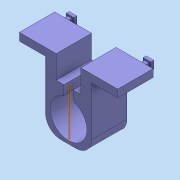
# Autodesk Inventor part: support_codeur
Saved by Autodesk Inventor 2017 (Build 210142000, 142)
## iProperties
Created: 2017-12-27
Part Number: support_codeur
Material: Generic
Document SubType Name: Modeling
Designer: franc
Density: 1 g/cm^3
Appearance: Default
Author: franc
Autodesk Inventor part; units mm, degrees
ref_plane "YZ Plane" through (0, 0, 0) normal (1, 0, 0) x (0, 1, 0)
ref_plane "XZ Plane" through (0, 0, 0) normal (0, 1, 0) x (-1, 0, 0)
ref_plane "XY Plane" through (0, 0, 0) normal (0, 0, 1) x (1, 0, 0)
sketch "Esquisse1" plane through (0, 0, 0) normal (0, 1, 0) x (-1, 0, 0)
  line L0 (7.2872, 10.2128) -> (-22.7128, 10.2128)
  line L1 (-22.7128, 10.2128) -> (-22.7128, -19.7872)
  line L2 (-22.7128, -19.7872) -> (7.2872, -19.7872)
  line L3 (7.2872, -19.7872) -> (7.2872, 10.2128)
  point P0 (0, 0)
  dimension "d0" = 30
  dimension "d1" = 30
  constraints: 8 end point, 2 parallel, 1 horizontal, 1 perpendicular
  measures "d0" distance of L2.end L0.start
  measures "d1" distance of L0.start L0.end
extrude "Extrusion1" add sketch "Esquisse1" along normal blind 23
ref_plane "Plan médian" through (7.7128, 0, 10.2128) normal (1, 0, 0) x (0, 0, -1)
sketch "Esquisse4" plane through (0, 0, 0) normal (0, -1, 0) x (1, 0, 0)
  circle A0 centre (7.7128, -7.8122) radius 11.975 projected
  arc A1 (4.2482, 4.1575) -> (4.0453, 3.779) centre (4.3314, 3.8692) ccw projected
  line L0 (4.1002, 3.6049) -> (4.0453, 3.779)
  line L1 (4.7128, 6.1957) -> (4.7128, 4.2818)
  arc A2 (11.3803, 3.779) -> (11.1773, 4.1575) centre (11.0942, 3.8692) ccw projected
  line L2 (11.3254, 3.6049) -> (11.3803, 3.779)
  line L3 (4.2482, 4.1575) -> (4.7128, 4.2781)
  line L4 (11.1773, 4.1575) -> (10.7128, 4.3039)
  line L5 (4.7128, 4.2818) -> (4.7128, 4.2781)
  line L6 (4.7128, 6.1957) -> (4.7128, 10.2128)
  line L7 (-7.2872, 10.2128) -> (22.7128, 10.2128) projected
  line L8 (10.7128, 5.8358) -> (10.7128, 10.2128)
  line L9 (10.7128, 5.8358) -> (10.7128, 4.3039)
  point P0 (0, 0)
  constraints: 18 end point, 5 point on line, 4 vertical, 3 point on circle, 1 parallel, 6 other
extrude "Extrusion2" cut sketch "Esquisse4" against normal blind 22
sketch "Esquisse5" plane through (0, 22, 0) normal (0, -1, 0) x (1, 0, 0)
  circle A0 centre (15.507, -3.3122) radius 1.25 projected
  circle A1 centre (-0.0815, -3.3122) radius 1.25 projected
  circle A2 centre (7.7128, -16.8122) radius 1.25 projected
  circle A3 centre (7.7128, -7.8122) radius 6 projected
  point P0 (0, 0)
extrude "Extrusion3" cut sketch "Esquisse5" against normal through all
sketch "Esquisse6" plane through (-7.2872, 23, 10.2128) normal (0, 0, 1) x (1, 0, 0)
  line L0 (0, -23) -> (12, -23) projected
  line L1 (5.9558, 0) -> (8.4558, 0) projected
  line L2 (0, -23) -> (7, -23)
  line L3 (7, -23) -> (7, 0)
  line L4 (7, 0) -> (0, 0)
  line L5 (0, 0) -> (0, -23)
  line L6 (30, -23) -> (30, 0) projected
  line L7 (0, 0) -> (30, 0) projected
  line L8 (30, -23) -> (23, -23)
  line L9 (23, -23) -> (23, 0)
  line L10 (23, 0) -> (30, 0)
  line L11 (30, 0) -> (30, -23)
  point P0 (7.2872, -23)
  dimension "d8" = 7
  dimension "d9" = 7
  constraints: 16 end point, 4 parallel, 2 horizontal, 2 perpendicular, 2 point on line
  measures "d8" distance between parallel lines of L5 L3
  measures "d9" distance between parallel lines of L6 L9
extrude "Extrusion4" add sketch "Esquisse6" along normal blind 10
sketch "Esquisse7" plane through (-7.2872, 23, 20.2128) normal (0, 0, 1) x (1, 0, 0)
  line L0 (7, 0) -> (-17, 0)
  line L1 (-17, 0) -> (-17, -23)
  line L2 (-17, -23) -> (7, -23)
  line L3 (7, -23) -> (7, 0)
  line L4 (30, 0) -> (0, 0) projected
  line L5 (23, 0) -> (47, 0)
  line L6 (47, 0) -> (47, -23)
  line L7 (47, -23) -> (23, -23)
  line L8 (23, -23) -> (23, 0)
  line L9 (0, 0) -> (0, -23) projected
  line L10 (30, -23) -> (30, 0) projected
  point P0 (7.2872, -23)
  dimension "d12" = 17
  dimension "d13" = 17
  constraints: 16 end point, 4 parallel, 2 horizontal, 2 perpendicular, 1 point on line
  measures "d12" distance between parallel lines of L1 L9
  measures "d13" distance between parallel lines of L6 L10
extrude "Extrusion5" add sketch "Esquisse7" along normal blind 5
sketch "Esquisse8" plane through (0, 23, 0) normal (0, 1, 0) x (1, 0, 0)
  line L0 (34.2128, -24.2128) -> (31.2128, -24.2128)
  line L1 (31.2128, -24.2128) -> (31.2128, -21.2128)
  line L2 (31.2128, -21.2128) -> (34.2128, -21.2128)
  line L3 (34.2128, -21.2128) -> (34.2128, -24.2128)
  line L4 (39.7128, -20.2128) -> (39.7128, -25.2128) projected
  line L5 (39.7128, -20.2128) -> (22.7128, -20.2128) projected
  line L6 (-16.0084, -24.2128) -> (-18.7872, -24.2128)
  line L7 (-18.7872, -24.2128) -> (-18.7872, -21.2128)
  line L8 (-18.7872, -21.2128) -> (-16.0084, -21.2128)
  line L9 (-16.0084, -21.2128) -> (-16.0084, -24.2128)
  line L10 (-0.2872, -25.2128) -> (-24.2872, -25.2128) projected
  line L11 (-24.2872, -20.2128) -> (-24.2872, -25.2128) projected
  point P0 (0, 0)
  point P1 (-0.4939, -25.2128)
  dimension "d16" = 5.5
  dimension "d17" = 3
  dimension "d18" = 3
  dimension "d19" = 1
  dimension "d20" = 3
  dimension "d21" = 1
  dimension "d22" = 5.5
  constraints: 16 end point, 4 parallel, 2 horizontal, 2 perpendicular
  measures "d16" distance between parallel lines of L4 L3
  measures "d17" distance of L2.end L0.start
  measures "d18" distance of L0.start L0.end
  measures "d19" distance between parallel lines of L5 L2
  measures "d20" distance of L6.end L7.end
  measures "d21" distance between parallel lines of L10 L6
  measures "d22" distance between parallel lines of L11 L7
extrude "Extrusion6" add sketch "Esquisse8" along normal blind 3
sketch "Esquisse9" plane through (0, 26, 0) normal (0, 1, 0) x (1, 0, 0)
  line L0 (15.7128, -25.2128) -> (39.7128, -25.2128) projected
  line L1 (22.7128, -20.2128) -> (39.7128, -20.2128) projected
  line L2 (35.2128, -25.2128) -> (30.2128, -25.2128)
  line L3 (30.2128, -25.2128) -> (30.2128, -20.2128)
  line L4 (30.2128, -20.2128) -> (35.2128, -20.2128)
  line L5 (35.2128, -20.2128) -> (35.2128, -25.2128)
  line L6 (39.7128, -20.2128) -> (39.7128, -25.2128) projected
  line L7 (-24.2872, -25.2128) -> (-0.2872, -25.2128) projected
  line L8 (-14.7872, -25.2128) -> (-19.7872, -25.2128)
  line L9 (-19.7872, -25.2128) -> (-19.7872, -20.2128)
  line L10 (-19.7872, -20.2128) -> (-14.7872, -20.2128)
  line L11 (-14.7872, -20.2128) -> (-14.7872, -25.2128)
  line L12 (-24.2872, -20.2128) -> (-24.2872, -25.2128) projected
  point P0 (0, 0)
  dimension "d25" = 5
  dimension "d26" = 4.5
  dimension "d27" = 4.5
  dimension "d28" = 5
  constraints: 16 end point, 4 parallel, 3 point on line, 2 horizontal, 2 perpendicular
  measures "d25" distance between parallel lines of L3 L5
  measures "d26" distance between parallel lines of L6 L5
  measures "d27" distance between parallel lines of L12 L9
  measures "d28" distance of L9.end L10.end
extrude "Extrusion7" add sketch "Esquisse9" along normal blind 2 contours L3 L1 L5 L0 | L9 L10 L11 L7
sketch "Esquisse10" plane through (22.7128, 23, -19.7872) normal (0, 0, -1) x (-1, 0, 0)
  line L0 (0, -23) -> (15, -23) projected
  line L1 (15, -23) -> (15, -1) projected
  line L2 (15, -23) -> (30, -23) projected
  line L3 (30, -23) -> (30, 0) projected
  line L4 (0, 0) -> (30, 0) projected
  line L5 (0, -23) -> (0, 0) projected
  line L6 (0, 0) -> (30, 0)
  line L7 (30, 0) -> (30, -23)
  line L8 (30, -23) -> (0, -23)
  line L9 (0, -23) -> (0, 0)
  point P0 (22.7128, -23)
  constraints: 8 end point, 2 parallel, 1 horizontal, 1 perpendicular
extrude "Extrusion8" add sketch "Esquisse10" along normal blind 2
fillet "Congé1" radius 10 2 edges at (22.7128, 11.5, -21.7872) (-7.2872, 11.5, -21.7872)
